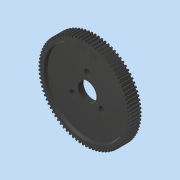
# Autodesk Inventor part: pistonSpurGear
Saved by Autodesk Inventor 2017 (Build 210142000, 142)
## iProperties
Created: 2016-11-28
Part Number: pistonSpurGear
Material: ABS Plastic
Document SubType Name: Modeling
Designer: techn
Density: 1.06 g/cm^3
Appearance: Smooth - Black
Author: techn
Autodesk Inventor part; units mm, degrees
ref_plane "YZ Plane" through (0, 0, 0) normal (1, 0, 0) x (0, 1, 0)
ref_plane "XZ Plane" through (0, 0, 0) normal (0, 1, 0) x (-1, 0, 0)
ref_plane "XY Plane" through (0, 0, 0) normal (0, 0, 1) x (1, 0, 0)
sketch "Sketch1" plane through (0, 0, 0) normal (0, 0, 1) x (1, 0, 0)
  circle A0 centre (0, 0) radius 21.844
  dimension "d0" = 43.688
  constraints: 1 centre point, 1 coincident
  measures "d0" diameter of A0
extrude "Extrusion1" add sketch "Sketch1" along normal blind 5.6642
sketch "Sketch2" plane through (0, 0, 0) normal (0, 0, -1) x (-1, 0, 0)
  line L0 (0, 0) -> (0, 8.3295)
  circle A0 centre (0, 8.3295) radius 1.5875
  circle A1 centre (-7.2136, -4.1648) radius 1.5875
  circle A2 centre (7.2136, -4.1648) radius 1.5875
  dimension "d3" = 3.175
  dimension "d6" = 360
  dimension "d8" = 14.4272
  constraints: 3 centre point, 2 end point, 1 coincident, 1 vertical, 7 other
  measures "d3" diameter of A0
  measures "d8" distance of A2.centre L0.end
extrude "Extrusion2" cut sketch "Sketch2" against normal through all
sketch "Sketch3" plane through (0, 0, 5.6642) normal (0, 0, 1) x (1, 0, 0)
  circle A0 centre (0, 0) radius 4.7625
  dimension "d11" = 9.525
  constraints: 1 centre point, 1 coincident
  measures "d11" diameter of A0
extrude "Extrusion3" cut sketch "Sketch3" against normal through all
sketch "Sketch4" plane through (0, 0, 5.6642) normal (0, 0, 1) x (1, 0, 0)
  line L0 (-0.2667, 22.8061) -> (0.2667, 22.8061)
  line L1 (0.2667, 22.8061) -> (0.3683, 22.2219)
  line L2 (0.3683, 22.2219) -> (0.3683, 21.8409)
  line L3 (0.3683, 21.8409) -> (-0.3683, 21.8409)
  line L4 (-0.3683, 21.8409) -> (-0.3683, 22.2219)
  line L5 (-0.3683, 22.2219) -> (-0.2667, 22.8061)
  circle A0 centre (0, 0) radius 21.844 construction
  point P0 (0, 22.8061)
  dimension "d14" = 0.5334
  dimension "d15" = 0.7366
  dimension "d16" = 0.9652
  dimension "d17" = 0.381
  constraints: 12 end point, 2 equal length, 2 perpendicular, 1 horizontal, 1 midpoint, 1 vertical, 1 vertical alignment, 2 other
  measures "d14" distance of L0.start L0.end
  measures "d15" distance of L2.end L3.end
  measures "d16" distance between parallel lines of L0 L3
  measures "d17" distance of L3.end L4.end
extrude "Extrusion4" add sketch "Sketch4" against normal up to surface (5.6642 mm away)
pattern_circular "Circular Pattern1" count 85 over 360 about axis through (0, 0, 0) along (0, 0, 1) of "Extrusion4"
sketch "Sketch6" plane through (0, 0, 5.6642) normal (0, 0, 1) x (1, 0, 0)
  circle A0 centre (0, 0) radius 19.685
  dimension "d25" = 39.37
  constraints: 1 centre point, 1 coincident
  measures "d25" diameter of A0
extrude "Extrusion5" cut sketch "Sketch6" against normal blind 1.397
chamfer "Chamfer1" distance 0.635 distance2 1.397 1 edges at (-19.685, 0, 5.6642) measured on face at (-20.185, 0, 5.6642)
sketch "Sketch7" plane through (0, 0, 0) normal (0, 0, -1) x (-1, 0, 0)
  circle A0 centre (0, 0) radius 19.685
  dimension "d31" = 39.37
  constraints: 1 centre point, 1 coincident
  measures "d31" diameter of A0
extrude "Extrusion6" cut sketch "Sketch7" against normal blind 1.397
chamfer "Chamfer2" distance 0.635 distance2 1.397 1 edges at (19.685, 0, 0) measured on face at (20.185, 0, 0)
sketch "Sketch8" plane through (0, 0, 4.2672) normal (0, 0, 1) x (1, 0, 0)
  line L0 (-6.0049, 17.9216) -> (5.7737, 17.9216) construction
  line L1 (5.7737, 17.9216) -> (5.7737, 15.4553) construction
  line L2 (5.7737, 15.4553) -> (-6.0049, 15.4553) construction
  line L3 (-6.0049, 15.4553) -> (-6.0049, 17.9216) construction
  spline S0 degree 2 poles (-5.1197, 15.4553) (-5.2956, 15.4553) (-5.5843, 15.5605) (-5.6856, 15.658) knots 0 0 0 1 2 2 2
  spline S1 degree 2 poles (-5.6856, 15.658) (-5.785, 15.7536) (-5.8882, 16.0136) (-5.8882, 16.1608) knots 0 0 0 1 2 2 2
  spline S2 degree 2 poles (-5.8882, 16.1608) (-5.8882, 16.352) (-5.6837, 16.6732) (-5.4887, 16.7687) knots 0 0 0 1 2 2 2
  line L4 (-5.4887, 16.7687) -> (-5.4887, 16.7783)
  spline S3 degree 2 poles (-5.4887, 16.7783) (-5.6626, 16.8796) (-5.8309, 17.1205) (-5.8309, 17.3002) knots 0 0 0 1 2 2 2
  spline S4 degree 2 poles (-5.8309, 17.3002) (-5.8309, 17.566) (-5.4294, 17.9216) (-5.1197, 17.9216) knots 0 0 0 1 2 2 2
  spline S5 degree 2 poles (-5.1197, 17.9216) (-4.7985, 17.9216) (-4.4104, 17.5851) (-4.4104, 17.3213) knots 0 0 0 1 2 2 2
  spline S6 degree 2 poles (-4.4104, 17.3213) (-4.4104, 17.1626) (-4.5959, 16.8529) (-4.7698, 16.7649) knots 0 0 0 1 2 2 2
  line L5 (-4.7698, 16.7649) -> (-4.7698, 16.7554)
  spline S7 degree 2 poles (-4.7698, 16.7554) (-4.5634, 16.6598) (-4.3512, 16.3845) (-4.3512, 16.1665) knots 0 0 0 1 2 2 2
  spline S8 degree 2 poles (-4.3512, 16.1665) (-4.3512, 15.8645) (-4.7909, 15.4553) (-5.1197, 15.4553) knots 0 0 0 1 2 2 2
  spline S9 degree 2 poles (-4.6762, 16.1359) (-4.6762, 16.2812) (-4.7909, 16.4533) (-4.9534, 16.5412) knots 0 0 0 1 2 2 2
  spline S10 degree 2 poles (-4.9534, 16.5412) (-5.0069, 16.5718) (-5.1866, 16.6426) (-5.2994, 16.6885) knots 0 0 0 1 2 2 2
  spline S11 degree 2 poles (-5.2994, 16.6885) (-5.4294, 16.6024) (-5.569, 16.3462) (-5.569, 16.1837) knots 0 0 0 1 2 2 2
  spline S12 degree 2 poles (-5.569, 16.1837) (-5.569, 15.9696) (-5.3109, 15.6905) (-5.1159, 15.6905) knots 0 0 0 1 2 2 2
  spline S13 degree 2 poles (-5.1159, 15.6905) (-4.917, 15.6905) (-4.6762, 15.9295) (-4.6762, 16.1359) knots 0 0 0 1 2 2 2
  spline S14 degree 2 poles (-4.7201, 17.3174) (-4.7201, 17.4761) (-4.9323, 17.6883) (-5.1216, 17.6883) knots 0 0 0 1 2 2 2
  spline S15 degree 2 poles (-5.1216, 17.6883) (-5.2937, 17.6883) (-5.5135, 17.4991) (-5.5135, 17.3366) knots 0 0 0 1 2 2 2
  spline S16 degree 2 poles (-5.5135, 17.3366) (-5.5135, 17.2199) (-5.4007, 17.0574) (-5.2879, 16.9924) knots 0 0 0 1 2 2 2
  spline S17 degree 2 poles (-5.2879, 16.9924) (-5.2401, 16.9657) (-5.0375, 16.872) (-4.9553, 16.8452) knots 0 0 0 1 2 2 2
  spline S18 degree 2 poles (-4.9553, 16.8452) (-4.8176, 16.9504) (-4.7201, 17.174) (-4.7201, 17.3174) knots 0 0 0 1 2 2 2
  spline S19 degree 2 poles (-2.6325, 16.2583) (-2.6325, 16.0882) (-2.7414, 15.7976) (-2.8408, 15.6905) knots 0 0 0 1 2 2 2
  spline S20 degree 2 poles (-2.8408, 15.6905) (-2.9403, 15.5834) (-3.2366, 15.4592) (-3.4201, 15.4592) knots 0 0 0 1 2 2 2
  spline S21 degree 2 poles (-3.4201, 15.4592) (-3.5883, 15.4592) (-3.9172, 15.5337) (-4.0376, 15.593) knots 0 0 0 1 2 2 2
  line L6 (-4.0376, 15.593) -> (-4.0376, 15.9276)
  line L7 (-4.0376, 15.9276) -> (-4.0147, 15.9276)
  spline S22 degree 2 poles (-4.0147, 15.9276) (-3.9784, 15.9008) (-3.8426, 15.832) (-3.7604, 15.8014) knots 0 0 0 1 2 2 2
  spline S23 degree 2 poles (-3.7604, 15.8014) (-3.6667, 15.7689) (-3.5119, 15.7326) (-3.4144, 15.7326) knots 0 0 0 1 2 2 2
  spline S24 degree 2 poles (-3.4144, 15.7326) (-3.3188, 15.7326) (-3.1391, 15.8014) (-3.0741, 15.8759) knots 0 0 0 1 2 2 2
  spline S25 degree 2 poles (-3.0741, 15.8759) (-3.0148, 15.9467) (-2.9536, 16.134) (-2.9536, 16.2602) knots 0 0 0 1 2 2 2
  spline S26 degree 2 poles (-2.9536, 16.2602) (-2.9536, 16.3864) (-3.0225, 16.547) (-3.0875, 16.6005) knots 0 0 0 1 2 2 2
  spline S27 degree 2 poles (-3.0875, 16.6005) (-3.1544, 16.6598) (-3.3532, 16.7095) (-3.4736, 16.7095) knots 0 0 0 1 2 2 2
  spline S28 degree 2 poles (-3.4736, 16.7095) (-3.6036, 16.7095) (-3.8617, 16.6693) (-3.9401, 16.6521) knots 0 0 0 1 2 2 2
  line L8 (-3.9401, 16.6521) -> (-3.9401, 17.868)
  line L9 (-3.9401, 17.868) -> (-2.6458, 17.868)
  line L10 (-2.6458, 17.868) -> (-2.6458, 17.5908)
  line L11 (-2.6458, 17.5908) -> (-3.6361, 17.5908)
  line L12 (-3.6361, 17.5908) -> (-3.6361, 16.9618)
  spline S29 degree 2 poles (-3.6361, 16.9618) (-3.5788, 16.9695) (-3.4679, 16.9752) (-3.422, 16.9752) knots 0 0 0 1 2 2 2
  spline S30 degree 2 poles (-3.422, 16.9752) (-3.2404, 16.9752) (-2.99, 16.916) (-2.8753, 16.828) knots 0 0 0 1 2 2 2
  spline S31 degree 2 poles (-2.8753, 16.828) (-2.7586, 16.7401) (-2.6325, 16.4724) (-2.6325, 16.2583) knots 0 0 0 1 2 2 2
  line L13 (-1.6746, 15.5089) -> (-1.6746, 17.5889)
  line L14 (-1.6746, 17.5889) -> (-2.4661, 17.5889)
  line L15 (-2.4661, 17.5889) -> (-2.4661, 17.868)
  line L16 (-2.4661, 17.868) -> (-0.5696, 17.868)
  line L17 (-0.5696, 17.868) -> (-0.5696, 17.5889)
  line L18 (-0.5696, 17.5889) -> (-1.3611, 17.5889)
  line L19 (-1.3611, 17.5889) -> (-1.3611, 15.5089)
  line L20 (-1.3611, 15.5089) -> (-1.6746, 15.5089)
  line L21 (2.1336, 16.3195) -> (1.8526, 16.3195)
  line L22 (1.8526, 16.3195) -> (1.8526, 15.5089)
  line L23 (1.8526, 15.5089) -> (1.5486, 15.5089)
  line L24 (1.5486, 15.5089) -> (1.5486, 16.3195)
  line L25 (1.5486, 16.3195) -> (0.5067, 16.3195)
  line L26 (0.5067, 16.3195) -> (0.5067, 16.6521)
  line L27 (0.5067, 16.6521) -> (1.562, 17.868)
  line L28 (1.562, 17.868) -> (1.8526, 17.868)
  line L29 (1.8526, 17.868) -> (1.8526, 16.5737)
  line L30 (1.8526, 16.5737) -> (2.1336, 16.5737)
  line L31 (2.1336, 16.5737) -> (2.1336, 16.3195)
  line L32 (1.5486, 16.5737) -> (1.5486, 17.4952)
  line L33 (1.5486, 17.4952) -> (0.7552, 16.5737)
  line L34 (0.7552, 16.5737) -> (1.5486, 16.5737)
  spline S32 degree 2 poles (3.0991, 15.4553) (2.9232, 15.4553) (2.6345, 15.5605) (2.5332, 15.658) knots 0 0 0 1 2 2 2
  spline S33 degree 2 poles (2.5332, 15.658) (2.4338, 15.7536) (2.3306, 16.0136) (2.3306, 16.1608) knots 0 0 0 1 2 2 2
  spline S34 degree 2 poles (2.3306, 16.1608) (2.3306, 16.352) (2.5351, 16.6732) (2.7301, 16.7687) knots 0 0 0 1 2 2 2
  line L35 (2.7301, 16.7687) -> (2.7301, 16.7783)
  spline S35 degree 2 poles (2.7301, 16.7783) (2.5562, 16.8796) (2.3879, 17.1205) (2.3879, 17.3002) knots 0 0 0 1 2 2 2
  spline S36 degree 2 poles (2.3879, 17.3002) (2.3879, 17.566) (2.7894, 17.9216) (3.0991, 17.9216) knots 0 0 0 1 2 2 2
  spline S37 degree 2 poles (3.0991, 17.9216) (3.4203, 17.9216) (3.8084, 17.5851) (3.8084, 17.3213) knots 0 0 0 1 2 2 2
  spline S38 degree 2 poles (3.8084, 17.3213) (3.8084, 17.1626) (3.6229, 16.8529) (3.449, 16.7649) knots 0 0 0 1 2 2 2
  line L36 (3.449, 16.7649) -> (3.449, 16.7554)
  spline S39 degree 2 poles (3.449, 16.7554) (3.6554, 16.6598) (3.8676, 16.3845) (3.8676, 16.1665) knots 0 0 0 1 2 2 2
  spline S40 degree 2 poles (3.8676, 16.1665) (3.8676, 15.8645) (3.4279, 15.4553) (3.0991, 15.4553) knots 0 0 0 1 2 2 2
  spline S41 degree 2 poles (3.5426, 16.1359) (3.5426, 16.2812) (3.4279, 16.4533) (3.2654, 16.5412) knots 0 0 0 1 2 2 2
  spline S42 degree 2 poles (3.2654, 16.5412) (3.2119, 16.5718) (3.0322, 16.6426) (2.9194, 16.6885) knots 0 0 0 1 2 2 2
  spline S43 degree 2 poles (2.9194, 16.6885) (2.7894, 16.6024) (2.6498, 16.3462) (2.6498, 16.1837) knots 0 0 0 1 2 2 2
  spline S44 degree 2 poles (2.6498, 16.1837) (2.6498, 15.9696) (2.9079, 15.6905) (3.1029, 15.6905) knots 0 0 0 1 2 2 2
  spline S45 degree 2 poles (3.1029, 15.6905) (3.3018, 15.6905) (3.5426, 15.9295) (3.5426, 16.1359) knots 0 0 0 1 2 2 2
  spline S46 degree 2 poles (3.4987, 17.3174) (3.4987, 17.4761) (3.2865, 17.6883) (3.0972, 17.6883) knots 0 0 0 1 2 2 2
  spline S47 degree 2 poles (3.0972, 17.6883) (2.9251, 17.6883) (2.7053, 17.4991) (2.7053, 17.3366) knots 0 0 0 1 2 2 2
  spline S48 degree 2 poles (2.7053, 17.3366) (2.7053, 17.2199) (2.8181, 17.0574) (2.9309, 16.9924) knots 0 0 0 1 2 2 2
  spline S49 degree 2 poles (2.9309, 16.9924) (2.9787, 16.9657) (3.1813, 16.872) (3.2635, 16.8452) knots 0 0 0 1 2 2 2
  spline S50 degree 2 poles (3.2635, 16.8452) (3.4012, 16.9504) (3.4987, 17.174) (3.4987, 17.3174) knots 0 0 0 1 2 2 2
  spline S51 degree 2 poles (5.7144, 17.1568) (5.7144, 17.0039) (5.6055, 16.7286) (5.508, 16.633) knots 0 0 0 1 2 2 2
  spline S52 degree 2 poles (5.508, 16.633) (5.3856, 16.5126) (5.0549, 16.3883) (4.8025, 16.3883) knots 0 0 0 1 2 2 2
  line L37 (4.8025, 16.3883) -> (4.5368, 16.3883)
  line L38 (4.5368, 16.3883) -> (4.5368, 15.5089)
  line L39 (4.5368, 15.5089) -> (4.2232, 15.5089)
  line L40 (4.2232, 15.5089) -> (4.2232, 17.868)
  line L41 (4.2232, 17.868) -> (4.8159, 17.868)
  spline S53 degree 2 poles (4.8159, 17.868) (5.0262, 17.868) (5.3206, 17.7992) (5.4334, 17.7208) knots 0 0 0 1 2 2 2
  spline S54 degree 2 poles (5.4334, 17.7208) (5.5653, 17.631) (5.7144, 17.3538) (5.7144, 17.1568) knots 0 0 0 1 2 2 2
  spline S55 degree 2 poles (5.3875, 17.1473) (5.3875, 17.2696) (5.3034, 17.4493) (5.2174, 17.5067) knots 0 0 0 1 2 2 2
  spline S56 degree 2 poles (5.2174, 17.5067) (5.1428, 17.5564) (4.944, 17.5966) (4.7968, 17.5966) knots 0 0 0 1 2 2 2
  line L42 (4.7968, 17.5966) -> (4.5368, 17.5966)
  line L43 (4.5368, 17.5966) -> (4.5368, 16.656)
  line L44 (4.5368, 16.656) -> (4.7509, 16.656)
  spline S57 degree 2 poles (4.7509, 16.656) (4.9421, 16.656) (5.1772, 16.7171) (5.2537, 16.7974) knots 0 0 0 1 2 2 2
  spline S58 degree 2 poles (5.2537, 16.7974) (5.3244, 16.8682) (5.3875, 17.0345) (5.3875, 17.1473) knots 0 0 0 1 2 2 2
  point P0 (0, 0)
  constraints: 2 other
emboss "Emboss2" sketch "Sketch8" operation cut depth 0.254 direction (0, 0, -1)
body "Solid1"
